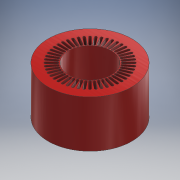
# Autodesk Inventor part: Stator
Saved by Autodesk Inventor 2018 (Build 220112000, 112)
## iProperties
Created: 2017-07-21
Part Number: Stator
Material: Типовые
Document SubType Name: Modeling
Designer: user
Density: 1 g/cm^3
Appearance: По умолчанию
Author: user
Autodesk Inventor part; units mm, degrees
ref_plane "YZ Plane" through (0, 0, 0) normal (1, 0, 0) x (0, 1, 0)
ref_plane "XZ Plane" through (0, 0, 0) normal (0, 1, 0) x (-1, 0, 0)
ref_plane "XY Plane" through (0, 0, 0) normal (0, 0, 1) x (1, 0, 0)
sketch "Эскиз1" plane through (0, 0, 0) normal (0, 0, 1) x (1, 0, 0)
  circle A0 centre (0, 0) radius 90.075
  circle A1 centre (0, 0) radius 177.75
  constraints: 2 centre point
extrude "Выдавливание1" add sketch "Эскиз1" against normal blind 200
sketch "Эскиз2" plane through (0, 0, 0) normal (0, 0, 1) x (1, 0, 0)
  arc A0 (97.375, 4.8) -> (97.375, -4.8) centre (97.375, 0) ccw
  line L0 (97.375, -4.8) -> (134.775, -4.8)
  arc A1 (134.775, -4.8) -> (134.775, 4.8) centre (134.775, 0) ccw
  line L1 (134.775, 4.8) -> (97.375, 4.8)
  constraints: 4 end point, 4 point on circle, 2 centre point
extrude "Выдавливание2" cut sketch "Эскиз2" against normal blind 200
pattern_circular "Круговой массив1" count 48 over 360 about axis through (0, 0, -10) along (0, 0, -1) of "Выдавливание2"
